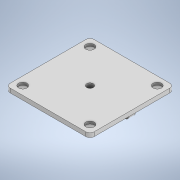
# Autodesk Inventor part: sliding_platform
Saved by Autodesk Inventor 2022 (Build 260153000, 153)
## iProperties
Created: 2021-07-07
Part Number: sliding_platform
Material: Generic
Document SubType Name: Modeling
Designer: fraaw
Density: 1 g/cm^3
Appearance: Default
Author: fraaw
## iProperties of the stored document sliding_platform_3DPrint.ipt
Created: 2021-07-07
Part Number: sliding_platform_3DPrint
Material: Generic
Document SubType Name: Modeling
Designer: fraaw
Density: 1 g/cm^3
Appearance: Default
Author: fraaw
Autodesk Inventor part; units mm, degrees
ref_plane "YZ Plane" through (0, 0, 0) normal (1, 0, 0) x (0, 1, 0)
ref_plane "XZ Plane" through (0, 0, 0) normal (0, 1, 0) x (-1, 0, 0)
ref_plane "XY Plane" through (0, 0, 0) normal (0, 0, 1) x (1, 0, 0)
sketch "Sketch1" plane through (0, 0, 0) normal (0, 1, 0) x (-1, 0, 0)
  line L0 (-50, -50) -> (50, -50)
  line L1 (50, -50) -> (50, 50)
  line L2 (50, 50) -> (-50, 50)
  line L3 (-50, 50) -> (-50, -50)
  line L4 (-50, -50) -> (50, 50) construction
  line L5 (50, -50) -> (-50, 50) construction
  point P0 (0, 0)
  dimension "d0" = 100
  dimension "d1" = 100
  constraints: 12 end point, 2 midpoint, 2 parallel, 1 horizontal, 1 perpendicular
  measures "d0" distance of L2.end L0.start
  measures "d1" distance of L1.end L2.end
extrude "Extrusion1" add sketch "Sketch1" along normal blind 5
sketch "Sketch2" plane through (0, 0, 0) normal (0, -1, 0) x (1, 0, 0)
  line L0 (50, 50) -> (50, -50) projected
  line L1 (-50, -4) -> (50, -4)
  line L2 (50, -4) -> (50, 4)
  line L3 (50, 4) -> (-50, 4)
  line L4 (-50, 4) -> (-50, -4)
  line L5 (-50, -4) -> (50, 4) construction
  line L6 (50, -4) -> (-50, 4) construction
  point P0 (0, 0)
  dimension "d4" = 8
  constraints: 12 end point, 2 midpoint, 2 parallel, 1 horizontal, 1 perpendicular, 1 point on line
  measures "d4" distance of L3.end L1.start
extrude "Extrusion2" add sketch "Sketch2" along normal blind 4
sketch "Sketch3" plane through (0, 5, 0) normal (0, 1, 0) x (1, 0, 0)
  point P0 (0, 0)
  point P1 (0, 0)
  constraints: 1 coincident
hole "Hole1" at (0, 5, 0) direction (0, -1, 0) diameter 8 depth 9
fillet "Fillet1" radius 5 4 edges at (50, 2.5, 50) (50, 2.5, -50) (-50, 2.5, 50) (-50, 2.5, -50)
sketch "Sketch7" plane through (0, 5, 0) normal (0, 1, 0) x (1, 0, 0)
  line L0 (40, -40) -> (-40, -40) construction
  line L1 (-40, -40) -> (-40, 40) construction
  line L2 (-40, 40) -> (40, 40) construction
  line L3 (40, 40) -> (40, -40) construction
  circle A0 centre (0, 0) radius 4 construction
  line L4 (40, -40) -> (-40, 40) construction
  line L5 (-40, -40) -> (40, 40) construction
  dimension "d27" = 80
  dimension "d28" = 80
  constraints: 12 end point, 2 midpoint, 2 parallel, 1 horizontal, 1 perpendicular
  measures "d27" distance of L0.end L1.end
  measures "d28" distance of L0.start L0.end
hole "Hole2" at (-40, 5, 40) at (40, 5, -40) at (40, 5, 40) at (-40, 5, -40) direction (0, -1, 0) diameter 10 depth 3
fillet "Fillet2" radius 4 2 edges at (50, -4, 0) (-50, -4, 0)
body "Solid1"
